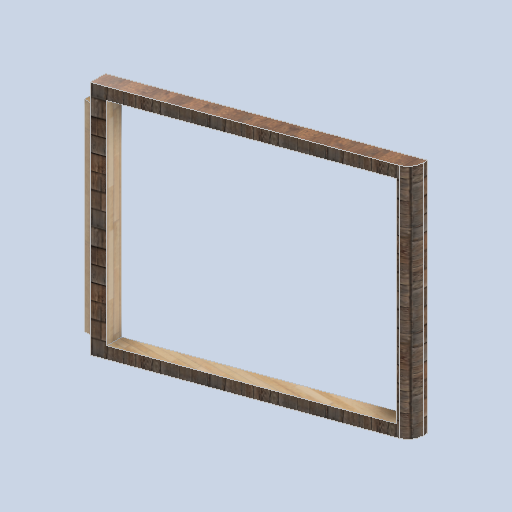
# Autodesk Inventor part: side_curve_frame_01
Saved by Autodesk Inventor 2024.2 (Build 282272000, 272)
## iProperties
Created: 2024-05-24
Part Number: side_curve_frame_01
Material: Wood (Maple)
Document SubType Name: Modeling
Designer: LOSTER_1
Density: 0.67 g/cm^3
Appearance: Natural Maple - Glossy Dark Tint
Author: LOSTER_1
Autodesk Inventor part; units mm, degrees
ref_plane "YZ Plane" through (0, 0, 0) normal (1, 0, 0) x (0, 1, 0)
ref_plane "XZ Plane" through (0, 0, 0) normal (0, 1, 0) x (-1, 0, 0)
sketch "Sketch1" plane through (0, 0, 0) normal (1, 0, 0) x (0, 1, 0)
  line L0 (-16080.1567, 1504.8391) -> (-13729.4879, 1504.8391)
  line L1 (-13729.4879, 1504.8391) -> (-13729.4879, 1354.8391)
  line L2 (-13729.4879, 1354.8391) -> (-16080.1567, 1354.8391)
  line L3 (-16080.1567, 1354.8391) -> (-16080.1567, 1504.8391)
  point P0 (0, 0)
  point P1 (-16255.1567, 1504.8391)
  point P2 (-15905.1567, 1504.8391)
  point P3 (-13904.4879, 1504.8391)
  point P4 (-13554.4879, 1504.8391)
  point P5 (-13729.4879, 1504.8391)
  dimension "d3" = 150
  constraints: 8 end point, 2 parallel, 1 horizontal, 1 perpendicular
  measures "d3" distance of L0.end L1.end
extrude "Extrusion1" add sketch "Sketch1" along normal blind 60
sketch "Sketch2" plane through (60, 0, 0) normal (1, 0, 0) x (0, 0, -1)
  line L0 (-1354.8391, -16080.1567) -> (-1354.8391, -13729.4879) projected
  line L1 (-1354.8391, -13729.4879) -> (-1504.8391, -13729.4879) projected
  line L2 (-1504.8391, -13729.4879) -> (-1504.8391, -16080.1567) projected
  line L3 (-1504.8391, -16080.1567) -> (-1354.8391, -16080.1567) projected
  point P0 (0, 0)
ref_plane "Work Plane1" through (0, -16080.1567, 1504.8391) normal (0, -1, 0) x (0, 0, -1)
sketch "Sketch3" plane through (0, -16080.1567, 1504.8391) normal (0, -1, 0) x (0, 0, -1)
  line L0 (0, 60) -> (150, 60) projected
  line L1 (0, 60) -> (150, 60)
  line L2 (0, 60) -> (855.0504, 2409.2316)
  line L3 (0, 60) -> (2500, 60) construction
  line L4 (150, 60) -> (1005.0504, 2409.2316)
  line L5 (150, 60) -> (2650, 60) construction
  line L6 (1005.0504, 2409.2316) -> (855.0504, 2409.2316)
  point P0 (1504.8391, 0)
  dimension "d6" = 2500
  dimension "d7" = 70
  dimension "d8" = 70
  constraints: 12 end point, 4 horizontal, 2 equal length
  measures "d6" distance of L0.start L2.end
  measures "d7" angle of L3 L2
  measures "d8" angle of L5 L4
extrude "Extrusion2" add sketch "Sketch3" against normal blind 2351
sketch "Sketch4" plane through (0, -16080.1567, 1504.8391) normal (0, 0, 1) x (1, 0, 0)
  line L0 (2409.2316, 0) -> (60, 0) projected
  line L1 (2409.2316, 0) -> (2409.2316, 2351) projected
  line L2 (60, 2351) -> (2409.2316, 2351) projected
  line L3 (60, 2350.6688) -> (60, 2351) projected
  line L4 (60, 2350.6688) -> (60, 0) projected
  line L5 (60, 2350.6688) -> (60, 0) projected
  line L6 (60, 0) -> (180, 0)
  line L7 (180, 0) -> (180, 120)
  line L8 (180, 120) -> (60, 120)
  line L9 (60, 120) -> (60, 0)
  line L10 (2409.2316, 2351) -> (2289.2316, 2351)
  line L11 (2289.2316, 2351) -> (2289.2316, 2231)
  line L12 (2289.2316, 2231) -> (2409.2316, 2231)
  line L13 (2409.2316, 2231) -> (2409.2316, 2351)
  line L14 (2289.2316, 2231) -> (180, 2231)
  line L15 (180, 2231) -> (180, 120)
  line L16 (180, 120) -> (2289.2316, 120)
  line L17 (2289.2316, 120) -> (2289.2316, 2231)
  point P0 (0, 16080.1567)
  dimension "d11" = 120
  dimension "d12" = 120
  dimension "d13" = 120
  dimension "d14" = 120
  constraints: 24 end point, 6 parallel, 3 horizontal, 3 perpendicular
  measures "d11" distance of L8.end L7.end
  measures "d12" distance of L7.end L6.end
  measures "d13" distance of L12.end L11.end
  measures "d14" distance of L11.end L10.end
extrude "Extrusion3" cut sketch "Sketch4" against normal through all contours L15 L14 L17 L16
fillet "Fillet1" radius 150 1 edges at (2409.2316, -14904.6567, 649.7888)
sketch "Sketch5" plane through (0, -16080.1567, 1504.8391) normal (0, 0, 1) x (1, 0, 0)
  line L0 (60, 0) -> (60, 2350.6688) projected
  line L1 (0, 175) -> (60, 175)
  line L2 (60, 175) -> (60, 0)
  line L3 (60, 0) -> (0, 0)
  line L4 (0, 0) -> (0, 175)
  line L5 (60, 2351) -> (2310.5346, 2351) projected
  line L6 (0, 2175.6688) -> (60, 2175.6688)
  line L7 (60, 2175.6688) -> (60, 2351)
  line L8 (60, 2351) -> (0, 2351)
  line L9 (0, 2351) -> (0, 2175.6688)
  point P0 (0, 16080.1567)
  constraints: 16 end point, 4 parallel, 2 horizontal, 2 perpendicular
extrude "Extrusion4" cut sketch "Sketch5" against normal through all
body "Solid1"
